Autodesk Fusion 360 part; units mm, degrees
note: some values were not read from the file. Chosen so that the rebuilt part matches the saved one: which face or edge a step refers to. Set by a fixed rule: which sketch regions a step uses.
(part 2 of 4)
sketch "Sketch13" plane through (0, 7, 0) normal (0, 1, 0) x (-1, 0, 0) in component "Button Base"
  line L0 (75.5, 17.1) -> (45.2, 17.1)
  line L1 (-81.5, 11.1) -> (-81.5, -11.1)
  line L2 (-75.5, -17.1) -> (-45.2, -17.1)
  line L3 (-42.2, -11.1) -> (-42.2, 11.1)
  circle A0 centre (-61.8, 12.9) radius 2.95
  circle A1 centre (-61.8, -12.9) radius 2.95
  circle A2 centre (-46.4, 0) radius 2.95
  circle A3 centre (-77.2, 0) radius 2.95
  line L4 (-73, 8.7) -> (-50.6, 8.7)
  line L5 (-50.6, 8.7) -> (-50.6, -8.7)
  line L6 (-50.6, -8.7) -> (-73, -8.7)
  line L7 (-73, -8.7) -> (-73, 8.7)
  circle A4 centre (-79.5, -15.1) radius 2
  circle A5 centre (-79.5, 15.1) radius 2
  line L8 (-81.5, -11.1) -> (-83.5, -11.1)
  line L9 (-83.5, -11.1) -> (-83.5, -19.1)
  line L10 (-83.5, -19.1) -> (-75.5, -19.1)
  line L11 (-75.5, -19.1) -> (-75.5, -17.1)
  line L12 (-75.5, 17.1) -> (-75.5, 19.1)
  line L13 (83.5, 19.1) -> (75.5, 19.1)
  line L14 (-83.5, 11.1) -> (-81.5, 11.1)
  line L15 (-45.2, -17.1) -> (-45.2, -19.1)
  line L16 (-45.2, -19.1) -> (-37.2, -19.1)
  line L17 (-37.2, -19.1) -> (-37.2, -17.1)
  line L18 (-37.2, -17.1) -> (-4, -17.1)
  line L19 (-4, -17.1) -> (-4, -19.1)
  line L20 (-4, -19.1) -> (4, -19.1)
  line L21 (4, -19.1) -> (4, -17.1)
  line L22 (4, -17.1) -> (37.2, -17.1)
  line L23 (37.2, -17.1) -> (37.2, -19.1)
  line L24 (37.2, -19.1) -> (45.2, -19.1)
  line L25 (45.2, -19.1) -> (45.2, -17.1)
  line L26 (45.2, -17.1) -> (75.5, -17.1)
  line L27 (75.5, -17.1) -> (75.5, -19.1)
  line L28 (75.5, -19.1) -> (83.5, -19.1)
  line L29 (83.5, -19.1) -> (83.5, -11.1)
  line L30 (83.5, -11.1) -> (81.5, -11.1)
  line L31 (81.5, -11.1) -> (81.5, 11.1)
  line L32 (81.5, 11.1) -> (83.5, 11.1)
  line L33 (83.5, 11.1) -> (83.5, 19.1)
  line L34 (75.5, 19.1) -> (75.5, 17.1)
  line L35 (45.2, 17.1) -> (45.2, 19.1)
  line L36 (45.2, 19.1) -> (37.2, 19.1)
  line L37 (37.2, 19.1) -> (37.2, 17.1)
  line L38 (37.2, 17.1) -> (4, 17.1)
  line L39 (4, 17.1) -> (4, 19.1)
  line L40 (4, 19.1) -> (-4, 19.1)
  line L41 (-4, 19.1) -> (-4, 17.1)
  line L42 (-4, 17.1) -> (-37.2, 17.1)
  line L43 (-37.2, 17.1) -> (-37.2, 19.1)
  line L44 (-37.2, 19.1) -> (-45.2, 19.1)
  line L45 (-45.2, 19.1) -> (-45.2, 17.1)
  line L46 (-45.2, 17.1) -> (-75.5, 17.1)
  line L47 (-1, -11.1) -> (-1, 11.1)
  line L48 (-1, 11.1) -> (1, 11.1)
  line L49 (1, 11.1) -> (1, -11.1)
  line L50 (1, -11.1) -> (-1, -11.1)
  line L51 (-42.2, 11.1) -> (-40.2, 11.1)
  line L52 (-40.2, 11.1) -> (-40.2, -11.1)
  line L53 (-40.2, -11.1) -> (-42.2, -11.1)
  circle A6 centre (-20.6, 12.9) radius 2.95
  circle A7 centre (36, 0) radius 2.95
  circle A8 centre (77.2, 0) radius 2.95
  circle A9 centre (61.8, -12.9) radius 2.95
  circle A10 centre (20.6, -12.9) radius 2.95
  circle A11 centre (-5.2, 0) radius 2.95
  circle A12 centre (-20.6, -12.9) radius 2.95
  circle A13 centre (20.6, 12.9) radius 2.95
  circle A14 centre (61.8, 12.9) radius 2.95
  circle A15 centre (46.4, 0) radius 2.95
  circle A16 centre (5.2, 0) radius 2.95
  circle A17 centre (-36, 0) radius 2.95
  line L54 (9.4, 8.7) -> (31.8, 8.7)
  line L55 (31.8, 8.7) -> (31.8, -8.7)
  line L56 (31.8, -8.7) -> (9.4, -8.7)
  line L57 (9.4, -8.7) -> (9.4, 8.7)
  line L58 (-31.8, 8.7) -> (-9.4, 8.7)
  line L59 (-9.4, 8.7) -> (-9.4, -8.7)
  line L60 (-9.4, -8.7) -> (-31.8, -8.7)
  line L61 (-31.8, -8.7) -> (-31.8, 8.7)
  line L62 (73, 8.7) -> (73, -8.7)
  line L63 (73, -8.7) -> (50.6, -8.7)
  line L64 (50.6, -8.7) -> (50.6, 8.7)
  line L65 (50.6, 8.7) -> (73, 8.7)
  line L66 (42.2, 11.1) -> (42.2, -11.1)
  line L67 (42.2, -11.1) -> (40.2, -11.1)
  line L68 (40.2, -11.1) -> (40.2, 11.1)
  line L69 (40.2, 11.1) -> (42.2, 11.1)
  circle A18 centre (-79.5, -15.1) radius 3.05
  circle A19 centre (-79.5, 15.1) radius 3.05
  line L70 (-75.5, 19.1) -> (-83.5, 19.1)
  line L71 (-83.5, 19.1) -> (-83.5, 11.1)
  line L72 (-83.5, 19.1) -> (-75.5, 19.1)
  line L73 (-83.5, 11.1) -> (-83.5, 19.1)
  dimension "d798" = 4
  dimension "d799" = 4
  dimension "d1564" = 4
  dimension "d1565" = 4
  constraint concentric A4 A18
  measures "d798" diameter of A5
  measures "d799" diameter of A4
  measures "d1564" distance of A5.centre L72
  measures "d1565" distance of A5.centre L73
sketch "Sketch8" plane through (0, 33, 0) normal (0, 1, 0) x (-1, 0, 0) in component "Box"
  line L0 (83.75, -21) -> (83.75, -11)
  line L1 (83.75, -11) -> (78.75, -11)
  line L2 (78.75, -11) -> (78.75, -21)
  line L3 (78.75, -21) -> (83.75, -21)
  circle A0 centre (79.75, -15) radius 2
  line L4 (-83.75, -26) -> (83.75, -26)
  line L5 (83.75, -26) -> (83.75, 26)
  line L6 (-83.5, 19.1) -> (83.5, 19.1)
  line L7 (83.5, 19.1) -> (83.5, -19.1)
  line L8 (83.5, -19.1) -> (-83.5, -19.1)
  line L9 (-83.5, -19.1) -> (-83.5, 19.1)
  line L10 (-83.5, 19.1) -> (83.5, -19.1) construction
  line L11 (83.5, 19.1) -> (-83.5, -19.1) construction
  line L12 (86.75, 29) -> (86.75, -29)
  circle A1 centre (79.75, 15) radius 2
  line L13 (83.75, 26) -> (-83.75, 26)
  line L14 (83.75, 11) -> (83.75, 21)
  line L15 (83.75, 21) -> (78.75, 21)
  line L16 (78.75, 21) -> (78.75, 11)
  line L17 (78.75, 11) -> (83.75, 11)
  circle A2 centre (-79.5, -15) radius 2
  circle A3 centre (-79.5, 15) radius 2
  line L18 (83.75, 26) -> (73.75, 26)
  circle A4 centre (-79.75, -24.8) radius 2
  line L19 (-73.75, 29) -> (-86.75, 29)
  line L20 (-86.75, 29) -> (-86.75, -29)
  line L21 (-86.75, -29) -> (86.75, -29)
  line L22 (86.75, -29) -> (86.75, 29)
  line L23 (86.75, 29) -> (83.75, 29)
  line L24 (83.75, 29) -> (83.75, 26)
  line L25 (73.75, 26) -> (73.75, 21)
  line L26 (73.75, 21) -> (83.75, 21)
  line L27 (83.75, 21) -> (83.75, -21)
  line L28 (83.75, -21) -> (73.75, -21)
  line L29 (73.75, -21) -> (73.75, -26)
  line L30 (73.75, -26) -> (-73.75, -26)
  line L31 (-73.75, -26) -> (-73.75, -21)
  line L32 (-73.75, -21) -> (-83.75, -21)
  line L33 (-83.75, -21) -> (-83.75, 21)
  line L34 (-83.75, 21) -> (-73.75, 21)
  line L35 (-73.75, 21) -> (-73.75, 29)
  circle A5 centre (79.75, -24.8) radius 2
  circle A6 centre (79.75, 24.8) radius 0.8915
  circle A7 centre (-79.75, 24.8) radius 0.8915
  dimension "d803" = 4
  dimension "d805" = 4
  dimension "d869" = 38.2
  dimension "d870" = 167
  dimension "d872" = 58
  dimension "d874" = 11
  dimension "d875" = 4
  dimension "d876" = 11
  dimension "d877" = 4
  dimension "d897" = 4
  dimension "d898" = 11
  dimension "d899" = 4
  dimension "d900" = 4
  dimension "d901" = 11
  constraint perpendicular L6 L7
  constraint parallel L6 L8
  constraint parallel L7 L9
  constraint horizontal L6
  constraint coincident L10 origin
  constraint coincident L11 origin
  constraint equal A2 A3
  measures "d803" diameter of A0
  measures "d805" distance of A0.centre L5
  measures "d869" distance of L6.end L7.end
  measures "d870" distance of L7.end L8.end
  measures "d872" distance of L12.start L12.end
  measures "d874" distance of A0.centre L4
  measures "d875" distance of L5 A1.centre
  measures "d876" distance of A1.centre L13
  measures "d877" diameter of A1
  measures "d897" diameter of A2
  measures "d898" distance of L4 A2.centre
  measures "d899" distance of L9 A2.centre
  measures "d900" distance of L9 A3.centre
  measures "d901" distance of L13 A3.centre
extrude "Extrude9'" [suppressed] in component "Button Base"
thread "Thread1'" [suppressed] in component "Button Base"
mirror "Mirror1'" [suppressed] in component "Button Base"
sketch "Sketch15" plane through (0, 7, 0) normal (0, 1, 0) x (-1, 0, 0) in component "Button Base"
mirror "Mirror7" [suppressed] in component "Box"
mirror "Mirror8" [suppressed] in component "Box"
extrude "Extrude10" [suppressed] in component "Box"
extrude "Extrude11" [suppressed] in component "Box"
thread "Thread2" [suppressed] in component "Box"
sketch "Sketch9" plane through (0, 0, 11) normal (0, 0, -1) x (-1, 0, 0) in component "Box"
  line L0 (-73.75, 21) -> (-83.75, 21)
  line L1 (-83.75, 21) -> (-83.75, 3)
  line L2 (-83.75, 3) -> (-73.75, 3)
  line L3 (-73.75, 3) -> (-73.75, 21)
sketch "Sketch10" plane through (0, 33, 0) normal (0, 1, 0) x (-1, 0, 0) in component "Button"
  line L0 (-78.2129, 54.1152) -> (-80.2129, 54.1152)
  line L1 (-80.2129, 54.1152) -> (-80.2129, 46.1152)
  line L2 (-80.2129, 46.1152) -> (-72.2129, 46.1152)
  line L3 (-72.2129, 46.1152) -> (-72.2129, 48.1152)
  line L4 (-72.2129, 48.1152) -> (-41.9129, 48.1152)
  line L5 (-41.9129, 48.1152) -> (-41.9129, 46.1152)
  line L6 (-41.9129, 46.1152) -> (-33.9129, 46.1152)
  line L7 (-33.9129, 46.1152) -> (-33.9129, 48.1152)
  line L8 (-33.9129, 48.1152) -> (-0.7129, 48.1152)
  line L9 (-0.7129, 48.1152) -> (-0.7129, 46.1152)
  line L10 (-0.7129, 46.1152) -> (7.2871, 46.1152)
  line L11 (7.2871, 46.1152) -> (7.2871, 48.1152)
  line L12 (7.2871, 48.1152) -> (40.4871, 48.1152)
  line L13 (40.4871, 48.1152) -> (40.4871, 46.1152)
  line L14 (40.4871, 46.1152) -> (48.4871, 46.1152)
  line L15 (48.4871, 46.1152) -> (48.4871, 48.1152)
  line L16 (48.4871, 48.1152) -> (78.7871, 48.1152)
  line L17 (78.7871, 48.1152) -> (78.7871, 46.1152)
  line L18 (78.7871, 46.1152) -> (86.7871, 46.1152)
  line L19 (86.7871, 46.1152) -> (86.7871, 54.1152)
  line L20 (86.7871, 54.1152) -> (84.7871, 54.1152)
  line L21 (84.7871, 54.1152) -> (84.7871, 76.3152)
  line L22 (84.7871, 76.3152) -> (86.7871, 76.3152)
  line L23 (86.7871, 76.3152) -> (86.7871, 84.3152)
  line L24 (86.7871, 84.3152) -> (78.7871, 84.3152)
  line L25 (78.7871, 84.3152) -> (78.7871, 82.3152)
  line L26 (78.7871, 82.3152) -> (48.4871, 82.3152)
  line L27 (48.4871, 82.3152) -> (48.4871, 84.3152)
  line L28 (48.4871, 84.3152) -> (40.4871, 84.3152)
  line L29 (40.4871, 84.3152) -> (40.4871, 82.3152)
  line L30 (40.4871, 82.3152) -> (7.2871, 82.3152)
  line L31 (7.2871, 82.3152) -> (7.2871, 84.3152)
  line L32 (7.2871, 84.3152) -> (-0.7129, 84.3152)
  line L33 (-0.7129, 84.3152) -> (-0.7129, 82.3152)
  line L34 (-0.7129, 82.3152) -> (-33.9129, 82.3152)
  line L35 (-33.9129, 82.3152) -> (-33.9129, 84.3152)
  line L36 (-33.9129, 84.3152) -> (-41.9129, 84.3152)
  line L37 (-41.9129, 84.3152) -> (-41.9129, 82.3152)
  line L38 (-41.9129, 82.3152) -> (-72.2129, 82.3152)
  line L39 (-72.2129, 82.3152) -> (-72.2129, 84.3152)
  line L40 (-72.2129, 84.3152) -> (-80.2129, 84.3152)
  line L41 (-80.2129, 76.3152) -> (-78.2129, 76.3152)
  line L42 (-78.2129, 76.3152) -> (-78.2129, 54.1152)
  line L43 (2.2871, 54.1152) -> (2.2871, 76.3152)
  line L44 (2.2871, 76.3152) -> (4.2871, 76.3152)
  line L45 (4.2871, 76.3152) -> (4.2871, 54.1152)
  line L46 (4.2871, 54.1152) -> (2.2871, 54.1152)
  line L47 (-38.9129, 54.1152) -> (-38.9129, 76.3152)
  line L48 (-38.9129, 76.3152) -> (-36.9129, 76.3152)
  line L49 (-36.9129, 76.3152) -> (-36.9129, 54.1152)
  line L50 (-36.9129, 54.1152) -> (-38.9129, 54.1152)
  circle A0 centre (-58.5129, 78.1152) radius 2.95
  circle A1 centre (-17.3129, 78.1152) radius 2.95
  circle A2 centre (39.2871, 65.2152) radius 2.95
  circle A3 centre (80.4871, 65.2152) radius 2.95
  circle A4 centre (65.0871, 52.3152) radius 2.95
  circle A5 centre (23.8871, 52.3152) radius 2.95
  circle A6 centre (-1.9129, 65.2152) radius 2.95
  circle A7 centre (-58.5129, 52.3152) radius 2.95
  circle A8 centre (-43.1129, 65.2152) radius 2.95
  circle A9 centre (-17.3129, 52.3152) radius 2.95
  circle A10 centre (23.8871, 78.1152) radius 2.95
  circle A11 centre (65.0871, 78.1152) radius 2.95
  circle A12 centre (49.6871, 65.2152) radius 2.95
  circle A13 centre (8.4871, 65.2152) radius 2.95
  circle A14 centre (-32.7129, 65.2152) radius 2.95
  circle A15 centre (-73.9129, 65.2152) radius 2.95
  line L51 (12.6871, 73.9152) -> (35.0871, 73.9152)
  line L52 (35.0871, 73.9152) -> (35.0871, 56.5152)
  line L53 (35.0871, 56.5152) -> (12.6871, 56.5152)
  line L54 (12.6871, 56.5152) -> (12.6871, 73.9152)
  line L55 (-28.5129, 73.9152) -> (-6.1129, 73.9152)
  line L56 (-6.1129, 73.9152) -> (-6.1129, 56.5152)
  line L57 (-6.1129, 56.5152) -> (-28.5129, 56.5152)
  line L58 (-28.5129, 56.5152) -> (-28.5129, 73.9152)
  line L59 (76.2871, 73.9152) -> (76.2871, 56.5152)
  line L60 (76.2871, 56.5152) -> (53.8871, 56.5152)
  line L61 (53.8871, 56.5152) -> (53.8871, 73.9152)
  line L62 (53.8871, 73.9152) -> (76.2871, 73.9152)
  line L63 (-69.7129, 73.9152) -> (-47.3129, 73.9152)
  line L64 (-47.3129, 73.9152) -> (-47.3129, 56.5152)
  line L65 (-47.3129, 56.5152) -> (-69.7129, 56.5152)
  line L66 (-69.7129, 56.5152) -> (-69.7129, 73.9152)
  line L67 (45.4871, 76.3152) -> (45.4871, 54.1152)
  line L68 (45.4871, 54.1152) -> (43.4871, 54.1152)
  line L69 (43.4871, 54.1152) -> (43.4871, 76.3152)
  line L70 (43.4871, 76.3152) -> (45.4871, 76.3152)
  circle A16 centre (65.0871, 78.1152) radius 2.95
  circle A17 centre (49.6871, 65.2152) radius 2.95
  circle A18 centre (65.0871, 52.3152) radius 2.95
  circle A19 centre (80.4871, 65.2152) radius 2.95
  line L71 (-80.2129, 84.3152) -> (-80.2129, 76.3152)
  circle A20 centre (-76.2129, 50.1152) radius 3.05
  circle A21 centre (-76.2129, 80.3152) radius 3.05
  circle A22 centre (82.7871, 80.3152) radius 3.05
  circle A23 centre (82.7871, 50.1152) radius 3.05
sketch "Sketch5 (3)" plane through (-3.2871, 24.0807, 65.2152) normal (0, 1, 0) x (-1, 0, 0) in component "Button"
  line L0 (-81.5, -11.1) -> (-83.5, -11.1)
  line L1 (-83.5, -11.1) -> (-83.5, -19.1)
  line L2 (-83.5, -19.1) -> (-75.5, -19.1)
  line L3 (-75.5, -19.1) -> (-75.5, -17.1)
  line L4 (-75.5, -17.1) -> (-45.2, -17.1)
  line L5 (-45.2, -17.1) -> (-45.2, -19.1)
  line L6 (-45.2, -19.1) -> (-37.2, -19.1)
  line L7 (-37.2, -19.1) -> (-37.2, -17.1)
  line L8 (-37.2, -17.1) -> (-4, -17.1)
  line L9 (-4, -17.1) -> (-4, -19.1)
  line L10 (-4, -19.1) -> (4, -19.1)
  line L11 (4, -19.1) -> (4, -17.1)
  line L12 (4, -17.1) -> (37.2, -17.1)
  line L13 (37.2, -17.1) -> (37.2, -19.1)
  line L14 (37.2, -19.1) -> (45.2, -19.1)
  line L15 (45.2, -19.1) -> (45.2, -17.1)
  line L16 (45.2, -17.1) -> (75.5, -17.1)
  line L17 (75.5, -17.1) -> (75.5, -19.1)
  line L18 (75.5, -19.1) -> (83.5, -19.1)
  line L19 (83.5, -19.1) -> (83.5, -11.1)
  line L20 (83.5, -11.1) -> (81.5, -11.1)
  line L21 (81.5, -11.1) -> (81.5, 11.1)
  line L22 (81.5, 11.1) -> (83.5, 11.1)
  line L23 (83.5, 11.1) -> (83.5, 19.1)
  line L24 (83.5, 19.1) -> (75.5, 19.1)
  line L25 (75.5, 19.1) -> (75.5, 17.1)
  line L26 (75.5, 17.1) -> (45.2, 17.1)
  line L27 (45.2, 17.1) -> (45.2, 19.1)
  line L28 (45.2, 19.1) -> (37.2, 19.1)
  line L29 (37.2, 19.1) -> (37.2, 17.1)
  line L30 (37.2, 17.1) -> (4, 17.1)
  line L31 (4, 17.1) -> (4, 19.1)
  line L32 (4, 19.1) -> (-4, 19.1)
  line L33 (-4, 19.1) -> (-4, 17.1)
  line L34 (-4, 17.1) -> (-37.2, 17.1)
  line L35 (-37.2, 17.1) -> (-37.2, 19.1)
  line L36 (-37.2, 19.1) -> (-45.2, 19.1)
  line L37 (-45.2, 19.1) -> (-45.2, 17.1)
  line L38 (-45.2, 17.1) -> (-75.5, 17.1)
  line L39 (-75.5, 17.1) -> (-75.5, 19.1)
  line L40 (-75.5, 19.1) -> (-83.5, 19.1)
  line L41 (-83.5, 11.1) -> (-81.5, 11.1)
  line L42 (-81.5, 11.1) -> (-81.5, -11.1)
  line L43 (-1, -11.1) -> (-1, 11.1)
  line L44 (-1, 11.1) -> (1, 11.1)
  line L45 (1, 11.1) -> (1, -11.1)
  line L46 (1, -11.1) -> (-1, -11.1)
  line L47 (-42.2, -11.1) -> (-42.2, 11.1)
  line L48 (-42.2, 11.1) -> (-40.2, 11.1)
  line L49 (-40.2, 11.1) -> (-40.2, -11.1)
  line L50 (-40.2, -11.1) -> (-42.2, -11.1)
  circle A0 centre (-61.8, 12.9) radius 2.95
  circle A1 centre (-20.6, 12.9) radius 2.95
  circle A2 centre (36, 0) radius 2.95
  circle A3 centre (77.2, 0) radius 2.95
  circle A4 centre (61.8, -12.9) radius 2.95
  circle A5 centre (20.6, -12.9) radius 2.95
  circle A6 centre (-5.2, 0) radius 2.95
  circle A7 centre (-61.8, -12.9) radius 2.95
  circle A8 centre (-46.4, 0) radius 2.95
  circle A9 centre (-20.6, -12.9) radius 2.95
  circle A10 centre (20.6, 12.9) radius 2.95
  circle A11 centre (61.8, 12.9) radius 2.95
  circle A12 centre (46.4, 0) radius 2.95
  circle A13 centre (5.2, 0) radius 2.95
  circle A14 centre (-36, 0) radius 2.95
  circle A15 centre (-77.2, 0) radius 2.95
  line L51 (9.4, 8.7) -> (31.8, 8.7)
  line L52 (31.8, 8.7) -> (31.8, -8.7)
  line L53 (31.8, -8.7) -> (9.4, -8.7)
  line L54 (9.4, -8.7) -> (9.4, 8.7)
  line L55 (-31.8, 8.7) -> (-9.4, 8.7)
  line L56 (-9.4, 8.7) -> (-9.4, -8.7)
  line L57 (-9.4, -8.7) -> (-31.8, -8.7)
  line L58 (-31.8, -8.7) -> (-31.8, 8.7)
  line L59 (73, 8.7) -> (73, -8.7)
  line L60 (73, -8.7) -> (50.6, -8.7)
  line L61 (50.6, -8.7) -> (50.6, 8.7)
  line L62 (50.6, 8.7) -> (73, 8.7)
  line L63 (-73, 8.7) -> (-50.6, 8.7)
  line L64 (-50.6, 8.7) -> (-50.6, -8.7)
  line L65 (-50.6, -8.7) -> (-73, -8.7)
  line L66 (-73, -8.7) -> (-73, 8.7)
  line L67 (42.2, 11.1) -> (42.2, -11.1)
  line L68 (42.2, -11.1) -> (40.2, -11.1)
  line L69 (40.2, -11.1) -> (40.2, 11.1)
  line L70 (40.2, 11.1) -> (42.2, 11.1)
  circle A16 centre (20.6, 12.9) radius 2.95
  line L71 (-1, -11.1) -> (1, -11.1)
  line L72 (1, -11.1) -> (1, 11.1)
  line L73 (1, 11.1) -> (-1, 11.1)
  line L74 (-1, 11.1) -> (-1, -11.1)
  circle A17 centre (20.6, -12.9) radius 2.95
  line L75 (4, -19.1) -> (37.2, -19.1)
  line L76 (37.2, -19.1) -> (37.2, -17.1)
  line L77 (37.2, -17.1) -> (4, -17.1)
  line L78 (4, -17.1) -> (4, -19.1)
  line L79 (42.2, 11.1) -> (40.2, 11.1)
  line L80 (40.2, 11.1) -> (40.2, -11.1)
  line L81 (40.2, -11.1) -> (42.2, -11.1)
  line L82 (42.2, -11.1) -> (42.2, 11.1)
  line L83 (37.2, 19.1) -> (4, 19.1)
  line L84 (4, 19.1) -> (4, 17.1)
  line L85 (4, 17.1) -> (37.2, 17.1)
  line L86 (37.2, 17.1) -> (37.2, 19.1)
  line L87 (39.6, -16.8333) -> (1.6, -16.8333)
  line L88 (1.6, -16.8333) -> (1.6, 16.6667)
  line L89 (1.6, 16.6667) -> (39.6, 16.6667)
  line L90 (39.6, 16.6667) -> (39.6, -16.8333)
  line L91 (39.6, -16.8333) -> (1.6, 16.6667) construction
  line L92 (1.6, -16.8333) -> (39.6, 16.6667) construction
  line L93 (-83.5, 19.1) -> (-83.5, 11.1)
  circle A18 centre (-79.5, -15.1) radius 3.05
  circle A19 centre (-79.5, 15.1) radius 3.05
  circle A20 centre (79.5, 15.1) radius 3.05
  circle A21 centre (79.5, -15.1) radius 3.05
  point P0 (5.2, 0)
  point P1 (20.6, -12.9)
  point P2 (20.6, -0.0833)
  dimension "d849" = 38
  dimension "d850" = 33.5
  constraint perpendicular L87 L88
  constraint parallel L87 L89
  constraint parallel L88 L90
  constraint horizontal L87
  constraint coincident L91 P2
  constraint coincident L92 P2
  measures "d849" distance of L88.end L89.end
  measures "d850" distance of L87.end L88.end
extrude "Extrude5''" [suppressed] in component "Button"
sketch "Sketch7 (2)" plane through (0, 24.0807, 0) normal (0, 1, 0) x (-1, 0, 0) in component "Button"
  circle A0 centre (23.8871, 52.3152) radius 2.95
  circle A1 centre (23.8871, 78.1152) radius 2.95
  circle A2 centre (8.4871, 65.2152) radius 2.95
  circle A3 centre (39.2871, 65.2152) radius 2.95
  line L0 (42.8871, 81.8819) -> (4.8871, 81.8819)
  line L1 (4.8871, 81.8819) -> (4.8871, 48.3819)
  line L2 (4.8871, 48.3819) -> (42.8871, 48.3819)
  line L3 (42.8871, 48.3819) -> (42.8871, 81.8819)
  line L4 (42.8871, 48.3819) -> (4.8871, 48.3819)
  line L5 (4.8871, 48.3819) -> (4.8871, 81.8819)
  line L6 (4.8871, 81.8819) -> (42.8871, 81.8819)
  line L7 (42.8871, 81.8819) -> (42.8871, 48.3819)
  dimension "d859" = 38
  constraint horizontal L4
  constraint vertical L5
  constraint horizontal L6
  constraint vertical L7
  constraint coincident L0.end L1.start
  constraint coincident L2.end L3.start
  measures "d859" distance of L2.end L1.end
extrude "Extrude7" [suppressed] in component "Button"
sketch "Sketch8 (2)" plane through (0, 24.6807, 0) normal (0, 1, 0) x (-1, 0, 0) in component "Button"
  line L0 (42.8871, 81.8819) -> (4.8871, 81.8819)
  line L1 (4.8871, 81.8819) -> (4.8871, 48.3819)
  line L2 (4.8871, 48.3819) -> (42.8871, 48.3819)
  line L3 (42.8871, 48.3819) -> (42.8871, 81.8819)
  circle A0 centre (23.8871, 65.1319) radius 14
  dimension "d862" = 19
  dimension "d863" = 16.75
  dimension "d864" = 28
  dimension "d865" = 38
  dimension "d866" = 33.5
  measures "d862" distance of L1 A0.centre
  measures "d863" distance of L0 A0.centre
  measures "d864" diameter of A0
  measures "d865" distance of L1.end L2.end
  measures "d866" distance of L0.start L2.end
extrude "Extrude8'" [suppressed] in component "Button"
sketch "Sketch9 (2)" plane through (-4.8871, 0, 0) normal (1, 0, 0) x (0, 0, -1) in component "Button"
  line L0 (-81.8819, 24.6807) -> (-81.8819, 21.6807)
  line L1 (-81.8819, 21.6807) -> (-48.3819, 21.6807)
  line L2 (-48.3819, 21.6807) -> (-48.3819, 24.6807)
  line L3 (-48.3819, 24.6807) -> (-81.8819, 24.6807)
other "Base Feature1" in component "ButtonPink v5"
sketch "Sketch1 (5)" plane through (0, 45, 0) normal (0, 1, 0) x (-1, 0, 0) in component "ButtonPink v5"
  line L0 (-111.8498, 7.1011) -> (-111.8498, -10.2989)
  line L1 (-111.8498, -10.2989) -> (-134.2498, -10.2989)
  line L2 (-134.2498, -10.2989) -> (-134.2498, 7.1011)
  line L3 (-134.2498, 7.1011) -> (-111.8498, 7.1011)
  circle A0 centre (-138.4498, -1.5989) radius 3.1
  circle A1 centre (-123.0498, 11.3011) radius 3.1
  circle A2 centre (-123.0498, -14.4989) radius 3.1
  circle A3 centre (-107.6498, -1.5989) radius 3.1
  line L4 (-103.4498, -18.6989) -> (-103.4498, 15.5011)
  line L5 (-103.4498, 15.5011) -> (-142.6498, 15.5011)
  line L6 (-142.6498, 15.5011) -> (-142.6498, -18.6989)
  line L7 (-142.6498, -18.6989) -> (-103.4498, -18.6989)
  circle A4 centre (-138.4498, -1.5989) radius 3.1
  circle A5 centre (-123.0498, -14.4989) radius 3.1
  circle A6 centre (-107.6498, -1.5989) radius 3.1
  circle A7 centre (-123.0498, 11.3011) radius 3.1
  line L8 (-154.8498, 7.1011) -> (-154.8498, -10.2989)
  line L9 (-177.2498, -10.2989) -> (-177.2498, 7.1011)
  line L10 (-146.7095, 15.4507) -> (-185.4095, 15.5014)
  line L11 (-177.2498, 7.1011) -> (-154.8498, 7.1011)
  circle A8 centre (-166.0498, -14.4989) radius 3.1
  circle A9 centre (-181.4498, -1.5989) radius 3.1
  line L12 (-185.4095, 15.5014) -> (-185.4536, -18.1986)
  circle A10 centre (-181.4498, -1.5989) radius 3.1
  line L13 (-146.7537, -18.2493) -> (-146.7095, 15.4507)
  circle A11 centre (-166.0498, 11.3011) radius 3.1
  circle A12 centre (-166.0498, 11.3011) radius 3.1
  line L14 (-154.8498, -10.2989) -> (-177.2498, -10.2989)
  circle A13 centre (-150.6498, -1.5989) radius 3.1
  circle A14 centre (-150.6498, -1.5989) radius 3.1
  line L15 (-185.4536, -18.1986) -> (-146.7537, -18.2493)
  circle A15 centre (-166.0498, -14.4989) radius 3.1
  arc A16 (86.5, -27.2432) -> (86.5, -22.3568) centre (88.5, -24.8) ccw
  arc A17 (-86.5, -22.3568) -> (-86.5, -27.2432) centre (-88.5, -24.8) ccw
  line L16 (86.5, 29) -> (-86.5, 29)
  line L17 (-86.5, 29) -> (-86.5, 27.2432)
  line L18 (-86.5, -29) -> (86.5, -29)
  line L19 (86.5, -29) -> (86.5, -27.2432)
  arc A18 (86.5, 22.3568) -> (86.5, 27.2432) centre (88.5, 24.8) ccw
  arc A19 (-86.5, 27.2432) -> (-86.5, 22.3568) centre (-88.5, 24.8) ccw
  line L20 (-86.5, 22.3568) -> (-86.5, -22.3568)
  line L21 (-86.5, -27.2432) -> (-86.5, -29)
  line L22 (86.5, -22.3568) -> (86.5, 22.3568)
  line L23 (86.5, 27.2432) -> (86.5, 29)
  dimension "d623_3" = 39.2
  dimension "d624_3" = 38.7
  dimension "d625_3" = 33.7
  dimension "d921_3" = 0
  dimension "d922_3" = 0
  dimension "d923_3" = 0
  dimension "d924_3" = 0
  constraint perpendicular L12 L15
  constraint parallel L10 L15
  constraint parallel L12 L13
  measures "d623_3" distance of L4.start L6.end
  measures "d624_3" distance of L13.start L12.end
  measures "d625_3" vertical distance of L10.end L12.end
extrude "Extrude1'''" [suppressed] in component "ButtonPink v5"
sketch "Sketch2 (4)" plane through (0, 45, 0) normal (0, 1, 0) x (-1, 0, 0) in component "ButtonPink v5"
  line L0 (-142.6498, -18.6989) -> (-103.4498, -18.6989)
  line L1 (-103.4498, -18.6989) -> (-103.4498, 15.5011)
  line L2 (-103.4498, 15.5011) -> (-142.6498, 15.5011)
  line L3 (-142.6498, 15.5011) -> (-142.6498, -18.6989)
extrude "Extrude2''''" [suppressed] in component "ButtonPink v5"
sketch "Sketch3 (4)" plane through (0, 49.8, 0) normal (0, 1, 0) x (-1, 0, 0) in component "ButtonPink v5"
  line L0 (-142.6498, 15.5011) -> (-142.6498, -18.6989)
  line L1 (-142.6498, -18.6989) -> (-103.4498, -18.6989)
  line L2 (-103.4498, -18.6989) -> (-103.4498, 15.5011)
  line L3 (-103.4498, 15.5011) -> (-142.6498, 15.5011)
  circle A0 centre (-123.0498, -1.5989) radius 14
  dimension "d616_3" = 28
  dimension "d617_3" = 17.1
  dimension "d618_3" = 34.2
  dimension "d619_3" = 39.2
  dimension "d620_3" = 19.6
  measures "d616_3" diameter of A0
  measures "d617_3" distance of L1 A0.centre
  measures "d618_3" distance of L1 L3
  measures "d619_3" distance of L0 L2
  measures "d620_3" distance of L2 A0.centre
extrude "Extrude3'''" [suppressed] in component "ButtonPink v5"
sketch "Sketch4 (4)" plane through (0, 49.8, 0) normal (0, 1, 0) x (-1, 0, 0) in component "ButtonPink v5"
  circle A0 centre (-123.0498, -1.5989) radius 14
  line L0 (-142.6498, 15.5011) -> (-142.6498, -18.6989)
  line L1 (-142.6498, -18.6989) -> (-103.4498, -18.6989)
  line L2 (-103.4498, -18.6989) -> (-103.4498, 15.5011)
  line L3 (-103.4498, 15.5011) -> (-142.6498, 15.5011)
  line L4 (-103.9498, 15.0011) -> (-142.1498, 15.0011)
  line L5 (-142.1498, 15.0011) -> (-142.1498, -18.1989)
  line L6 (-142.1498, -18.1989) -> (-103.9498, -18.1989)
  line L7 (-103.9498, -18.1989) -> (-103.9498, 15.0011)
  dimension "d627_3" = -0.5
extrude "Extrude4'''" [suppressed] in component "ButtonPink v5"
sketch "Sketch10 (2)" plane through (0, 37.0807, 0) normal (0, 1, 0) x (-1, 0, 0) in component "ButtonPink v5"
  circle A0 centre (80.75, -16) radius 2.1574
  circle A1 centre (80.75, 16.2) radius 2.1574
  circle A2 centre (-80.25, -16) radius 2.1574
  circle A3 centre (-80.25, 16.2) radius 2.1574
  line L0 (-81.25, -11) -> (-83.25, -11)
  line L1 (-83.25, -11) -> (-83.25, -19)
  line L2 (-83.25, -19) -> (-75.25, -19)
  line L3 (-75.25, -19) -> (-75.25, -17)
  line L4 (-75.25, -17) -> (-44.95, -17)
  line L5 (-44.95, -17) -> (-44.95, -19)
  line L6 (-44.95, -19) -> (-36.95, -19)
  line L7 (-36.95, -19) -> (-36.95, -17)
  line L8 (-36.95, -17) -> (-3.75, -17)
  line L9 (-3.75, -17) -> (-3.75, -19)
  line L10 (-3.75, -19) -> (4.25, -19)
  line L11 (4.25, -19) -> (4.25, -17)
  line L12 (4.25, -17) -> (37.45, -17)
  line L13 (37.45, -17) -> (37.45, -19)
  line L14 (37.45, -19) -> (45.45, -19)
  line L15 (45.45, -19) -> (45.45, -17)
  line L16 (45.45, -17) -> (75.75, -17)
  line L17 (75.75, -17) -> (75.75, -19)
  line L18 (75.75, -19) -> (83.75, -19)
  line L19 (83.75, -19) -> (83.75, -11)
  line L20 (83.75, -11) -> (81.75, -11)
  line L21 (81.75, -11) -> (81.75, 11.2)
  line L22 (81.75, 11.2) -> (83.75, 11.2)
  line L23 (83.75, 11.2) -> (83.75, 19.2)
  line L24 (83.75, 19.2) -> (75.75, 19.2)
  line L25 (75.75, 19.2) -> (75.75, 17.2)
  line L26 (75.75, 17.2) -> (45.45, 17.2)
  line L27 (45.45, 17.2) -> (45.45, 19.2)
  line L28 (45.45, 19.2) -> (37.45, 19.2)
  line L29 (37.45, 19.2) -> (37.45, 17.2)
  line L30 (37.45, 17.2) -> (4.25, 17.2)
  line L31 (4.25, 17.2) -> (4.25, 19.2)
  line L32 (4.25, 19.2) -> (-3.75, 19.2)
  line L33 (-3.75, 19.2) -> (-3.75, 17.2)
  line L34 (-3.75, 17.2) -> (-36.95, 17.2)
  line L35 (-36.95, 17.2) -> (-36.95, 19.2)
  line L36 (-36.95, 19.2) -> (-44.95, 19.2)
  line L37 (-44.95, 19.2) -> (-44.95, 17.2)
  line L38 (-44.95, 17.2) -> (-75.25, 17.2)
  line L39 (-75.25, 17.2) -> (-75.25, 19.2)
  line L40 (-75.25, 19.2) -> (-83.25, 19.2)
  line L41 (-83.25, 19.2) -> (-83.25, 11.2)
  line L42 (-83.25, 11.2) -> (-81.25, 11.2)
  line L43 (-81.25, 11.2) -> (-81.25, -11)
  line L44 (-0.75, -11) -> (-0.75, 11.2)
  line L45 (-0.75, 11.2) -> (1.25, 11.2)
  line L46 (1.25, 11.2) -> (1.25, -11)
  line L47 (1.25, -11) -> (-0.75, -11)
  line L48 (-41.95, -11) -> (-41.95, 11.2)
  line L49 (-41.95, 11.2) -> (-39.95, 11.2)
  line L50 (-39.95, 11.2) -> (-39.95, -11)
  line L51 (-39.95, -11) -> (-41.95, -11)
  circle A4 centre (-61.55, 13) radius 3.1
  circle A5 centre (-20.35, 13) radius 3.1
  circle A6 centre (36.25, 0.1) radius 3.1
  circle A7 centre (77.45, 0.1) radius 3.1
  circle A8 centre (62.05, -12.8) radius 3.1
  circle A9 centre (20.85, -12.8) radius 3.1
  circle A10 centre (-4.95, 0.1) radius 3.1
  circle A11 centre (-61.55, -12.8) radius 3.1
  circle A12 centre (-46.15, 0.1) radius 3.1
  circle A13 centre (-20.35, -12.8) radius 3.1
  circle A14 centre (20.85, 13) radius 3.1
  circle A15 centre (62.05, 13) radius 3.1
  circle A16 centre (46.65, 0.1) radius 3.1
  circle A17 centre (5.45, 0.1) radius 3.1
  circle A18 centre (-35.75, 0.1) radius 3.1
  circle A19 centre (-76.95, 0.1) radius 3.1
  line L52 (9.65, 8.8) -> (32.05, 8.8)
  line L53 (32.05, 8.8) -> (32.05, -8.6)
  line L54 (32.05, -8.6) -> (9.65, -8.6)
  line L55 (9.65, -8.6) -> (9.65, 8.8)
  line L56 (-31.55, 8.8) -> (-9.15, 8.8)
  line L57 (-9.15, 8.8) -> (-9.15, -8.6)
  line L58 (-9.15, -8.6) -> (-31.55, -8.6)
  line L59 (-31.55, -8.6) -> (-31.55, 8.8)
  line L60 (73.25, 8.8) -> (73.25, -8.6)
  line L61 (73.25, -8.6) -> (50.85, -8.6)
  line L62 (50.85, -8.6) -> (50.85, 8.8)
  line L63 (50.85, 8.8) -> (73.25, 8.8)
  line L64 (-72.75, 8.8) -> (-50.35, 8.8)
  line L65 (-50.35, 8.8) -> (-50.35, -8.6)
  line L66 (-50.35, -8.6) -> (-72.75, -8.6)
  line L67 (-72.75, -8.6) -> (-72.75, 8.8)
  line L68 (42.45, 11.2) -> (42.45, -11)
  line L69 (42.45, -11) -> (40.45, -11)
  line L70 (40.45, -11) -> (40.45, 11.2)
  line L71 (40.45, 11.2) -> (42.45, 11.2)
  circle A20 centre (62.05, 13) radius 3.1
  circle A21 centre (46.65, 0.1) radius 3.1
  circle A22 centre (62.05, -12.8) radius 3.1
  circle A23 centre (77.45, 0.1) radius 3.1
sketch "Sketch5 (4)" plane through (0, 24.0807, 0) normal (0, 1, 0) x (-1, 0, 0) in component "ButtonPink v5"
  circle A0 centre (80.5, -16.1) radius 2.1574
  circle A1 centre (80.5, 16.1) radius 2.1574
  circle A2 centre (-80.5, -16.1) radius 2.1574
  circle A3 centre (-80.5, 16.1) radius 2.1574
  line L0 (-81.5, -11.1) -> (-83.5, -11.1)
  line L1 (-83.5, -11.1) -> (-83.5, -19.1)
  line L2 (-83.5, -19.1) -> (-75.5, -19.1)
  line L3 (-75.5, -19.1) -> (-75.5, -17.1)
  line L4 (-75.5, -17.1) -> (-45.2, -17.1)
  line L5 (-45.2, -17.1) -> (-45.2, -19.1)
  line L6 (-45.2, -19.1) -> (-37.2, -19.1)
  line L7 (-37.2, -19.1) -> (-37.2, -17.1)
  line L8 (-37.2, -17.1) -> (-4, -17.1)
  line L9 (-4, -17.1) -> (-4, -19.1)
  line L10 (-4, -19.1) -> (4, -19.1)
  line L11 (4, -19.1) -> (4, -17.1)
  line L12 (4, -17.1) -> (37.2, -17.1)
  line L13 (37.2, -17.1) -> (37.2, -19.1)
  line L14 (37.2, -19.1) -> (45.2, -19.1)
  line L15 (45.2, -19.1) -> (45.2, -17.1)
  line L16 (45.2, -17.1) -> (75.5, -17.1)
  line L17 (75.5, -17.1) -> (75.5, -19.1)
  line L18 (75.5, -19.1) -> (83.5, -19.1)
  line L19 (83.5, -19.1) -> (83.5, -11.1)
  line L20 (83.5, -11.1) -> (81.5, -11.1)
  line L21 (81.5, -11.1) -> (81.5, 11.1)
  line L22 (81.5, 11.1) -> (83.5, 11.1)
  line L23 (83.5, 11.1) -> (83.5, 19.1)
  line L24 (83.5, 19.1) -> (75.5, 19.1)
  line L25 (75.5, 19.1) -> (75.5, 17.1)
  line L26 (75.5, 17.1) -> (45.2, 17.1)
  line L27 (45.2, 17.1) -> (45.2, 19.1)
  line L28 (45.2, 19.1) -> (37.2, 19.1)
  line L29 (37.2, 19.1) -> (37.2, 17.1)
  line L30 (37.2, 17.1) -> (4, 17.1)
  line L31 (4, 17.1) -> (4, 19.1)
  line L32 (4, 19.1) -> (-4, 19.1)
  line L33 (-4, 19.1) -> (-4, 17.1)
  line L34 (-4, 17.1) -> (-37.2, 17.1)
  line L35 (-37.2, 17.1) -> (-37.2, 19.1)
  line L36 (-37.2, 19.1) -> (-45.2, 19.1)
  line L37 (-45.2, 19.1) -> (-45.2, 17.1)
  line L38 (-45.2, 17.1) -> (-75.5, 17.1)
  line L39 (-75.5, 17.1) -> (-75.5, 19.1)
  line L40 (-75.5, 19.1) -> (-83.5, 19.1)
  line L41 (-83.5, 19.1) -> (-83.5, 11.1)
  line L42 (-83.5, 11.1) -> (-81.5, 11.1)
  line L43 (-81.5, 11.1) -> (-81.5, -11.1)
  line L44 (-1, -11.1) -> (-1, 11.1)
  line L45 (-1, 11.1) -> (1, 11.1)
  line L46 (1, 11.1) -> (1, -11.1)
  line L47 (1, -11.1) -> (-1, -11.1)
  line L48 (-42.2, -11.1) -> (-42.2, 11.1)
  line L49 (-42.2, 11.1) -> (-40.2, 11.1)
  line L50 (-40.2, 11.1) -> (-40.2, -11.1)
  line L51 (-40.2, -11.1) -> (-42.2, -11.1)
  circle A4 centre (-61.8, 12.9) radius 3.1
  circle A5 centre (-20.6, 12.9) radius 3.1
  circle A6 centre (36, 0) radius 3.1
  circle A7 centre (77.2, 0) radius 3.1
  circle A8 centre (61.8, -12.9) radius 3.1
  circle A9 centre (20.6, -12.9) radius 3.1
  circle A10 centre (-5.2, 0) radius 3.1
  circle A11 centre (-61.8, -12.9) radius 3.1
  circle A12 centre (-46.4, 0) radius 3.1
  circle A13 centre (-20.6, -12.9) radius 3.1
  circle A14 centre (20.6, 12.9) radius 3.1
  circle A15 centre (61.8, 12.9) radius 3.1
  circle A16 centre (46.4, 0) radius 3.1
  circle A17 centre (5.2, 0) radius 3.1
  circle A18 centre (-36, 0) radius 3.1
  circle A19 centre (-77.2, 0) radius 3.1
  line L52 (9.4, 8.7) -> (31.8, 8.7)
  line L53 (31.8, 8.7) -> (31.8, -8.7)
  line L54 (31.8, -8.7) -> (9.4, -8.7)
  line L55 (9.4, -8.7) -> (9.4, 8.7)
  line L56 (-31.8, 8.7) -> (-9.4, 8.7)
  line L57 (-9.4, 8.7) -> (-9.4, -8.7)
  line L58 (-9.4, -8.7) -> (-31.8, -8.7)
  line L59 (-31.8, -8.7) -> (-31.8, 8.7)
  line L60 (73, 8.7) -> (73, -8.7)
  line L61 (73, -8.7) -> (50.6, -8.7)
  line L62 (50.6, -8.7) -> (50.6, 8.7)
  line L63 (50.6, 8.7) -> (73, 8.7)
  line L64 (-73, 8.7) -> (-50.6, 8.7)
  line L65 (-50.6, 8.7) -> (-50.6, -8.7)
  line L66 (-50.6, -8.7) -> (-73, -8.7)
  line L67 (-73, -8.7) -> (-73, 8.7)
  line L68 (42.2, 11.1) -> (42.2, -11.1)
  line L69 (42.2, -11.1) -> (40.2, -11.1)
  line L70 (40.2, -11.1) -> (40.2, 11.1)
  line L71 (40.2, 11.1) -> (42.2, 11.1)
  circle A20 centre (20.6, 12.9) radius 3.1
  line L72 (-1, -11.1) -> (1, -11.1)
  line L73 (1, -11.1) -> (1, 11.1)
  line L74 (1, 11.1) -> (-1, 11.1)
  line L75 (-1, 11.1) -> (-1, -11.1)
  circle A21 centre (20.6, -12.9) radius 3.1
  line L76 (4, -19.1) -> (37.2, -19.1)
  line L77 (37.2, -19.1) -> (37.2, -17.1)
  line L78 (37.2, -17.1) -> (4, -17.1)
  line L79 (4, -17.1) -> (4, -19.1)
  line L80 (42.2, 11.1) -> (40.2, 11.1)
  line L81 (40.2, 11.1) -> (40.2, -11.1)
  line L82 (40.2, -11.1) -> (42.2, -11.1)
  line L83 (42.2, -11.1) -> (42.2, 11.1)
  line L84 (37.2, 19.1) -> (4, 19.1)
  line L85 (4, 19.1) -> (4, 17.1)
  line L86 (4, 17.1) -> (37.2, 17.1)
  line L87 (37.2, 17.1) -> (37.2, 19.1)
  line L88 (39.6, -16.8333) -> (1.6, -16.8333)
  line L89 (1.6, -16.8333) -> (1.6, 16.6667)
  line L90 (1.6, 16.6667) -> (39.6, 16.6667)
  line L91 (39.6, 16.6667) -> (39.6, -16.8333)
  line L92 (39.6, -16.8333) -> (1.6, 16.6667) construction
  line L93 (1.6, -16.8333) -> (39.6, 16.6667) construction
  point P0 (5.2, 0)
  point P1 (20.6, -12.9)
  point P2 (20.6, -0.0833)
  dimension "d849_3" = 38
  dimension "d850_3" = 33.5
  constraint perpendicular L88 L89
  constraint parallel L88 L90
  constraint parallel L89 L91
  constraint horizontal L88
  constraint coincident L92 P2
  constraint coincident L93 P2
  measures "d849_3" distance of L89.end L90.end
  measures "d850_3" distance of L88.end L89.end
extrude "Extrude5'''" [suppressed] in component "ButtonPink v5"
sketch "Sketch7 (3)" plane through (0, 24.0807, 0) normal (0, 1, 0) x (-1, 0, 0) in component "ButtonPink v5"
  circle A0 centre (20.6, -12.9) radius 3.1
  circle A1 centre (20.6, 12.9) radius 3.1
  circle A2 centre (5.2, 0) radius 3.1
  circle A3 centre (36, 0) radius 3.1
  line L0 (39.6, 16.6667) -> (1.6, 16.6667)
  line L1 (1.6, 16.6667) -> (1.6, -16.8333)
  line L2 (1.6, -16.8333) -> (39.6, -16.8333)
  line L3 (39.6, -16.8333) -> (39.6, 16.6667)
  line L4 (39.6, -16.8333) -> (1.6, -16.8333)
  line L5 (1.6, -16.8333) -> (1.6, 16.6667)
  line L6 (1.6, 16.6667) -> (39.6, 16.6667)
  line L7 (39.6, 16.6667) -> (39.6, -16.8333)
  dimension "d859_3" = 38
  constraint horizontal L4
  constraint vertical L5
  constraint horizontal L6
  constraint vertical L7
  constraint coincident L0.end L1.start
  constraint coincident L2.end L3.start
  measures "d859_3" distance of L2.end L1.end
extrude "Extrude7'" [suppressed] in component "ButtonPink v5"
sketch "Sketch8 (3)" plane through (0, 25.2807, 0) normal (0, 1, 0) x (-1, 0, 0) in component "ButtonPink v5"
  line L0 (39.6, 16.6667) -> (1.6, 16.6667)
  line L1 (1.6, 16.6667) -> (1.6, -16.8333)
  line L2 (1.6, -16.8333) -> (39.6, -16.8333)
  line L3 (39.6, -16.8333) -> (39.6, 16.6667)
  circle A0 centre (20.6, -0.0833) radius 14
  dimension "d862_3" = 19
  dimension "d863_3" = 16.75
  dimension "d864_3" = 28
  dimension "d865_3" = 38
  dimension "d866_3" = 33.5
  measures "d862_3" distance of L1 A0.centre
  measures "d863_3" distance of L0 A0.centre
  measures "d864_3" diameter of A0
  measures "d865_3" distance of L1.end L2.end
  measures "d866_3" distance of L0.start L2.end
extrude "Extrude8''" [suppressed] in component "ButtonPink v5"
sketch "Sketch9 (3)" plane through (-1.6, 0, 0) normal (1, 0, 0) x (0, 0, -1) in component "ButtonPink v5"
  line L0 (-16.6667, 25.2807) -> (-16.6667, 22.2807)
  line L1 (-16.6667, 22.2807) -> (16.8333, 22.2807)
  line L2 (16.8333, 22.2807) -> (16.8333, 25.2807)
  line L3 (16.8333, 25.2807) -> (-16.6667, 25.2807)
other "Base Feature1'" in component "ButtonRed v5"
sketch "Sketch1 (6)" plane through (0, 45, 0) normal (0, 1, 0) x (-1, 0, 0) in component "ButtonRed v5"
  line L0 (-111.8498, 7.1011) -> (-111.8498, -10.2989)
  line L1 (-111.8498, -10.2989) -> (-134.2498, -10.2989)
  line L2 (-134.2498, -10.2989) -> (-134.2498, 7.1011)
  line L3 (-134.2498, 7.1011) -> (-111.8498, 7.1011)
  circle A0 centre (-138.4498, -1.5989) radius 3.1
  circle A1 centre (-123.0498, 11.3011) radius 3.1
  circle A2 centre (-123.0498, -14.4989) radius 3.1
  circle A3 centre (-107.6498, -1.5989) radius 3.1
  line L4 (-103.4498, -18.6989) -> (-103.4498, 15.5011)
  line L5 (-103.4498, 15.5011) -> (-142.6498, 15.5011)
  line L6 (-142.6498, 15.5011) -> (-142.6498, -18.6989)
  line L7 (-142.6498, -18.6989) -> (-103.4498, -18.6989)
  circle A4 centre (-138.4498, -1.5989) radius 3.1
  circle A5 centre (-123.0498, -14.4989) radius 3.1
  circle A6 centre (-107.6498, -1.5989) radius 3.1
  circle A7 centre (-123.0498, 11.3011) radius 3.1
  line L8 (-154.8498, 7.1011) -> (-154.8498, -10.2989)
  line L9 (-177.2498, -10.2989) -> (-177.2498, 7.1011)
  line L10 (-146.7095, 15.4507) -> (-185.4095, 15.5014)
  line L11 (-177.2498, 7.1011) -> (-154.8498, 7.1011)
  circle A8 centre (-166.0498, -14.4989) radius 3.1
  circle A9 centre (-181.4498, -1.5989) radius 3.1
  line L12 (-185.4095, 15.5014) -> (-185.4536, -18.1986)
  circle A10 centre (-181.4498, -1.5989) radius 3.1
  line L13 (-146.7537, -18.2493) -> (-146.7095, 15.4507)
  circle A11 centre (-166.0498, 11.3011) radius 3.1
  circle A12 centre (-166.0498, 11.3011) radius 3.1
  line L14 (-154.8498, -10.2989) -> (-177.2498, -10.2989)
  circle A13 centre (-150.6498, -1.5989) radius 3.1
  circle A14 centre (-150.6498, -1.5989) radius 3.1
  line L15 (-185.4536, -18.1986) -> (-146.7537, -18.2493)
  circle A15 centre (-166.0498, -14.4989) radius 3.1
  arc A16 (86.5, -27.2432) -> (86.5, -22.3568) centre (88.5, -24.8) ccw
  arc A17 (-86.5, -22.3568) -> (-86.5, -27.2432) centre (-88.5, -24.8) ccw
  line L16 (86.5, 29) -> (-86.5, 29)
  line L17 (-86.5, 29) -> (-86.5, 27.2432)
  line L18 (-86.5, -29) -> (86.5, -29)
  line L19 (86.5, -29) -> (86.5, -27.2432)
  arc A18 (86.5, 22.3568) -> (86.5, 27.2432) centre (88.5, 24.8) ccw
  arc A19 (-86.5, 27.2432) -> (-86.5, 22.3568) centre (-88.5, 24.8) ccw
  line L20 (-86.5, 22.3568) -> (-86.5, -22.3568)
  line L21 (-86.5, -27.2432) -> (-86.5, -29)
  line L22 (86.5, -22.3568) -> (86.5, 22.3568)
  line L23 (86.5, 27.2432) -> (86.5, 29)
  dimension "d623_2" = 39.2
  dimension "d624_2" = 38.7
  dimension "d625_2" = 33.7
  dimension "d921_2" = 0
  dimension "d922_2" = 0
  dimension "d923_2" = 0
  dimension "d924_2" = 0
  constraint perpendicular L12 L15
  constraint parallel L10 L15
  constraint parallel L12 L13
  measures "d623_2" distance of L4.start L6.end
  measures "d624_2" distance of L13.start L12.end
  measures "d625_2" vertical distance of L10.end L12.end
extrude "Extrude1''''" [suppressed] in component "ButtonRed v5"
sketch "Sketch2 (5)" plane through (0, 45, 0) normal (0, 1, 0) x (-1, 0, 0) in component "ButtonRed v5"
  line L0 (-142.6498, -18.6989) -> (-103.4498, -18.6989)
  line L1 (-103.4498, -18.6989) -> (-103.4498, 15.5011)
  line L2 (-103.4498, 15.5011) -> (-142.6498, 15.5011)
  line L3 (-142.6498, 15.5011) -> (-142.6498, -18.6989)
extrude "Extrude2'''''" [suppressed] in component "ButtonRed v5"
sketch "Sketch3 (5)" plane through (0, 49.8, 0) normal (0, 1, 0) x (-1, 0, 0) in component "ButtonRed v5"
  line L0 (-142.6498, 15.5011) -> (-142.6498, -18.6989)
  line L1 (-142.6498, -18.6989) -> (-103.4498, -18.6989)
  line L2 (-103.4498, -18.6989) -> (-103.4498, 15.5011)
  line L3 (-103.4498, 15.5011) -> (-142.6498, 15.5011)
  circle A0 centre (-123.0498, -1.5989) radius 14
  dimension "d616_2" = 28
  dimension "d617_2" = 17.1
  dimension "d618_2" = 34.2
  dimension "d619_2" = 39.2
  dimension "d620_2" = 19.6
  measures "d616_2" diameter of A0
  measures "d617_2" distance of L1 A0.centre
  measures "d618_2" distance of L1 L3
  measures "d619_2" distance of L0 L2
  measures "d620_2" distance of L2 A0.centre
extrude "Extrude3''''" [suppressed] in component "ButtonRed v5"
sketch "Sketch4 (5)" plane through (0, 49.8, 0) normal (0, 1, 0) x (-1, 0, 0) in component "ButtonRed v5"
  circle A0 centre (-123.0498, -1.5989) radius 14
  line L0 (-142.6498, 15.5011) -> (-142.6498, -18.6989)
  line L1 (-142.6498, -18.6989) -> (-103.4498, -18.6989)
  line L2 (-103.4498, -18.6989) -> (-103.4498, 15.5011)
  line L3 (-103.4498, 15.5011) -> (-142.6498, 15.5011)
  line L4 (-103.9498, 15.0011) -> (-142.1498, 15.0011)
  line L5 (-142.1498, 15.0011) -> (-142.1498, -18.1989)
  line L6 (-142.1498, -18.1989) -> (-103.9498, -18.1989)
  line L7 (-103.9498, -18.1989) -> (-103.9498, 15.0011)
  dimension "d627_2" = -0.5
extrude "Extrude4''''" [suppressed] in component "ButtonRed v5"
sketch "Sketch10 (3)" plane through (0, 37.0807, 0) normal (0, 1, 0) x (-1, 0, 0) in component "ButtonRed v5"
  circle A0 centre (80.75, -16) radius 2.1574
  circle A1 centre (80.75, 16.2) radius 2.1574
  circle A2 centre (-80.25, -16) radius 2.1574
  circle A3 centre (-80.25, 16.2) radius 2.1574
  line L0 (-81.25, -11) -> (-83.25, -11)
  line L1 (-83.25, -11) -> (-83.25, -19)
  line L2 (-83.25, -19) -> (-75.25, -19)
  line L3 (-75.25, -19) -> (-75.25, -17)
  line L4 (-75.25, -17) -> (-44.95, -17)
  line L5 (-44.95, -17) -> (-44.95, -19)
  line L6 (-44.95, -19) -> (-36.95, -19)
  line L7 (-36.95, -19) -> (-36.95, -17)
  line L8 (-36.95, -17) -> (-3.75, -17)
  line L9 (-3.75, -17) -> (-3.75, -19)
  line L10 (-3.75, -19) -> (4.25, -19)
  line L11 (4.25, -19) -> (4.25, -17)
  line L12 (4.25, -17) -> (37.45, -17)
  line L13 (37.45, -17) -> (37.45, -19)
  line L14 (37.45, -19) -> (45.45, -19)
  line L15 (45.45, -19) -> (45.45, -17)
  line L16 (45.45, -17) -> (75.75, -17)
  line L17 (75.75, -17) -> (75.75, -19)
  line L18 (75.75, -19) -> (83.75, -19)
  line L19 (83.75, -19) -> (83.75, -11)
  line L20 (83.75, -11) -> (81.75, -11)
  line L21 (81.75, -11) -> (81.75, 11.2)
  line L22 (81.75, 11.2) -> (83.75, 11.2)
  line L23 (83.75, 11.2) -> (83.75, 19.2)
  line L24 (83.75, 19.2) -> (75.75, 19.2)
  line L25 (75.75, 19.2) -> (75.75, 17.2)
  line L26 (75.75, 17.2) -> (45.45, 17.2)
  line L27 (45.45, 17.2) -> (45.45, 19.2)
  line L28 (45.45, 19.2) -> (37.45, 19.2)
  line L29 (37.45, 19.2) -> (37.45, 17.2)
  line L30 (37.45, 17.2) -> (4.25, 17.2)
  line L31 (4.25, 17.2) -> (4.25, 19.2)
  line L32 (4.25, 19.2) -> (-3.75, 19.2)
  line L33 (-3.75, 19.2) -> (-3.75, 17.2)
  line L34 (-3.75, 17.2) -> (-36.95, 17.2)
  line L35 (-36.95, 17.2) -> (-36.95, 19.2)
  line L36 (-36.95, 19.2) -> (-44.95, 19.2)
  line L37 (-44.95, 19.2) -> (-44.95, 17.2)
  line L38 (-44.95, 17.2) -> (-75.25, 17.2)
  line L39 (-75.25, 17.2) -> (-75.25, 19.2)
  line L40 (-75.25, 19.2) -> (-83.25, 19.2)
  line L41 (-83.25, 19.2) -> (-83.25, 11.2)
  line L42 (-83.25, 11.2) -> (-81.25, 11.2)
  line L43 (-81.25, 11.2) -> (-81.25, -11)
  line L44 (-0.75, -11) -> (-0.75, 11.2)
  line L45 (-0.75, 11.2) -> (1.25, 11.2)
  line L46 (1.25, 11.2) -> (1.25, -11)
  line L47 (1.25, -11) -> (-0.75, -11)
  line L48 (-41.95, -11) -> (-41.95, 11.2)
  line L49 (-41.95, 11.2) -> (-39.95, 11.2)
  line L50 (-39.95, 11.2) -> (-39.95, -11)
  line L51 (-39.95, -11) -> (-41.95, -11)
  circle A4 centre (-61.55, 13) radius 3.1
  circle A5 centre (-20.35, 13) radius 3.1
  circle A6 centre (36.25, 0.1) radius 3.1
  circle A7 centre (77.45, 0.1) radius 3.1
  circle A8 centre (62.05, -12.8) radius 3.1
  circle A9 centre (20.85, -12.8) radius 3.1
  circle A10 centre (-4.95, 0.1) radius 3.1
  circle A11 centre (-61.55, -12.8) radius 3.1
  circle A12 centre (-46.15, 0.1) radius 3.1
  circle A13 centre (-20.35, -12.8) radius 3.1
  circle A14 centre (20.85, 13) radius 3.1
  circle A15 centre (62.05, 13) radius 3.1
  circle A16 centre (46.65, 0.1) radius 3.1
  circle A17 centre (5.45, 0.1) radius 3.1
  circle A18 centre (-35.75, 0.1) radius 3.1
  circle A19 centre (-76.95, 0.1) radius 3.1
  line L52 (9.65, 8.8) -> (32.05, 8.8)
  line L53 (32.05, 8.8) -> (32.05, -8.6)
  line L54 (32.05, -8.6) -> (9.65, -8.6)
  line L55 (9.65, -8.6) -> (9.65, 8.8)
  line L56 (-31.55, 8.8) -> (-9.15, 8.8)
  line L57 (-9.15, 8.8) -> (-9.15, -8.6)
  line L58 (-9.15, -8.6) -> (-31.55, -8.6)
  line L59 (-31.55, -8.6) -> (-31.55, 8.8)
  line L60 (73.25, 8.8) -> (73.25, -8.6)
  line L61 (73.25, -8.6) -> (50.85, -8.6)
  line L62 (50.85, -8.6) -> (50.85, 8.8)
  line L63 (50.85, 8.8) -> (73.25, 8.8)
  line L64 (-72.75, 8.8) -> (-50.35, 8.8)
  line L65 (-50.35, 8.8) -> (-50.35, -8.6)
  line L66 (-50.35, -8.6) -> (-72.75, -8.6)
  line L67 (-72.75, -8.6) -> (-72.75, 8.8)
  line L68 (42.45, 11.2) -> (42.45, -11)
  line L69 (42.45, -11) -> (40.45, -11)
  line L70 (40.45, -11) -> (40.45, 11.2)
  line L71 (40.45, 11.2) -> (42.45, 11.2)
  circle A20 centre (62.05, 13) radius 3.1
  circle A21 centre (46.65, 0.1) radius 3.1
  circle A22 centre (62.05, -12.8) radius 3.1
  circle A23 centre (77.45, 0.1) radius 3.1